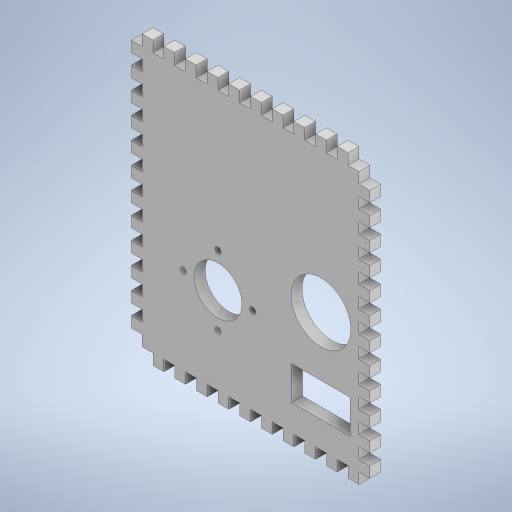
# Autodesk Inventor part: topside
Saved by Autodesk Inventor 2024 (Build 280153000, 153)
## iProperties
Created: 2024-04-15
Part Number: topside
Material: Generic
Document SubType Name: Modeling
Designer: srika
Density: 1 g/cm^3
Appearance: Default
Author: srika
Autodesk Inventor part; units mm, degrees
ref_plane "YZ Plane" through (0, 0, 0) normal (1, 0, 0) x (0, 1, 0)
ref_plane "XZ Plane" through (0, 0, 0) normal (0, 1, 0) x (-1, 0, 0)
ref_plane "XY Plane" through (0, 0, 0) normal (0, 0, 1) x (1, 0, 0)
sketch "Sketch1" plane through (0, 0, 0) normal (0, 0, 1) x (1, 0, 0)
  line L0 (5, 5) -> (105, 5)
  line L1 (105, 45) -> (105, 125)
  line L2 (105, 125) -> (5, 125)
  line L3 (5, 85) -> (5, 5)
  line L4 (0, 0) -> (5, 0)
  line L5 (5, 0) -> (5, 5)
  line L6 (5, 5) -> (0, 5)
  line L7 (0, 5) -> (0, 0)
  line L8 (105, 125) -> (110, 125)
  line L9 (110, 125) -> (110, 130)
  line L10 (110, 130) -> (105, 130)
  line L11 (105, 130) -> (105, 125)
  circle A0 centre (40, 45) radius 11
  circle A1 centre (24, 45) radius 1.4
  circle A2 centre (56, 45) radius 1.4
  circle A3 centre (40, 61) radius 1.4
  circle A4 centre (40, 29) radius 1.4
  circle A5 centre (87.5, 60) radius 13.7926
  line L12 (7.75, 7) -> (72.25, 7)
  line L13 (72.25, 7) -> (72.25, 83)
  line L14 (72.25, 83) -> (7.75, 83)
  line L15 (7.75, 83) -> (7.75, 7)
  line L16 (7.75, 7) -> (72.25, 83) construction
  line L17 (72.25, 7) -> (7.75, 83) construction
  line L18 (74, 17.25) -> (101, 17.25)
  line L19 (101, 17.25) -> (101, 32.75)
  line L20 (101, 32.75) -> (74, 32.75)
  line L21 (74, 32.75) -> (74, 17.25)
  line L22 (74, 17.25) -> (101, 32.75) construction
  line L23 (101, 17.25) -> (74, 32.75) construction
  line L24 (5, 125) -> (5, 85)
  line L25 (105, 45) -> (105, 5)
  line L26 (5, 15) -> (0, 15)
  line L27 (0, 10) -> (5, 10)
  line L28 (0, 15) -> (0, 10)
  line L29 (5, 10) -> (5, 15)
  line L30 (5, 25) -> (0, 25)
  line L31 (0, 20) -> (5, 20)
  line L32 (0, 25) -> (0, 20)
  line L33 (5, 20) -> (5, 25)
  line L34 (5, 35) -> (0, 35)
  line L35 (0, 30) -> (5, 30)
  line L36 (0, 35) -> (0, 30)
  line L37 (5, 30) -> (5, 35)
  line L38 (5, 45) -> (0, 45)
  line L39 (0, 40) -> (5, 40)
  line L40 (0, 45) -> (0, 40)
  line L41 (5, 40) -> (5, 45)
  line L42 (5, 55) -> (0, 55)
  line L43 (0, 50) -> (5, 50)
  line L44 (0, 55) -> (0, 50)
  line L45 (5, 50) -> (5, 55)
  line L46 (5, 65) -> (0, 65)
  line L47 (0, 60) -> (5, 60)
  line L48 (0, 65) -> (0, 60)
  line L49 (5, 60) -> (5, 65)
  line L50 (5, 75) -> (0, 75)
  line L51 (0, 70) -> (5, 70)
  line L52 (0, 75) -> (0, 70)
  line L53 (5, 70) -> (5, 75)
  line L54 (5, 85) -> (0, 85)
  line L55 (0, 80) -> (5, 80)
  line L56 (0, 85) -> (0, 80)
  line L57 (5, 80) -> (5, 85)
  line L58 (5, 95) -> (0, 95)
  line L59 (0, 90) -> (5, 90)
  line L60 (0, 95) -> (0, 90)
  line L61 (5, 90) -> (5, 95)
  line L62 (5, 105) -> (0, 105)
  line L63 (0, 100) -> (5, 100)
  line L64 (0, 105) -> (0, 100)
  line L65 (5, 100) -> (5, 105)
  line L66 (5, 115) -> (0, 115)
  line L67 (0, 110) -> (5, 110)
  line L68 (0, 115) -> (0, 110)
  line L69 (5, 110) -> (5, 115)
  line L70 (5, 125) -> (0, 125)
  line L71 (0, 120) -> (5, 120)
  line L72 (0, 125) -> (0, 120)
  line L73 (5, 120) -> (5, 125)
  line L74 (10, 0) -> (15, 0)
  line L75 (15, 0) -> (15, 5)
  line L76 (15, 5) -> (10, 5)
  line L77 (10, 5) -> (10, 0)
  line L78 (20, 0) -> (25, 0)
  line L79 (25, 0) -> (25, 5)
  line L80 (25, 5) -> (20, 5)
  line L81 (20, 5) -> (20, 0)
  line L82 (30, 0) -> (35, 0)
  line L83 (35, 0) -> (35, 5)
  line L84 (35, 5) -> (30, 5)
  line L85 (30, 5) -> (30, 0)
  line L86 (40, 0) -> (45, 0)
  line L87 (45, 0) -> (45, 5)
  line L88 (45, 5) -> (40, 5)
  line L89 (40, 5) -> (40, 0)
  line L90 (50, 0) -> (55, 0)
  line L91 (55, 0) -> (55, 5)
  line L92 (55, 5) -> (50, 5)
  line L93 (50, 5) -> (50, 0)
  line L94 (60, 0) -> (65, 0)
  line L95 (65, 0) -> (65, 5)
  line L96 (65, 5) -> (60, 5)
  line L97 (60, 5) -> (60, 0)
  line L98 (70, 0) -> (75, 0)
  line L99 (75, 0) -> (75, 5)
  line L100 (75, 5) -> (70, 5)
  line L101 (70, 5) -> (70, 0)
  line L102 (80, 0) -> (85, 0)
  line L103 (85, 0) -> (85, 5)
  line L104 (85, 5) -> (80, 5)
  line L105 (80, 5) -> (80, 0)
  line L106 (90, 0) -> (95, 0)
  line L107 (95, 0) -> (95, 5)
  line L108 (95, 5) -> (90, 5)
  line L109 (90, 5) -> (90, 0)
  line L110 (100, 0) -> (105, 0)
  line L111 (105, 0) -> (105, 5)
  line L112 (105, 5) -> (100, 5)
  line L113 (100, 5) -> (100, 0)
  line L114 (105, 120) -> (105, 115)
  line L115 (110, 120) -> (105, 120)
  line L116 (110, 115) -> (110, 120)
  line L117 (105, 115) -> (110, 115)
  line L118 (105, 110) -> (105, 105)
  line L119 (110, 110) -> (105, 110)
  line L120 (110, 105) -> (110, 110)
  line L121 (105, 105) -> (110, 105)
  line L122 (105, 100) -> (105, 95)
  line L123 (110, 100) -> (105, 100)
  line L124 (110, 95) -> (110, 100)
  line L125 (105, 95) -> (110, 95)
  line L126 (105, 90) -> (105, 85)
  line L127 (110, 90) -> (105, 90)
  line L128 (110, 85) -> (110, 90)
  line L129 (105, 85) -> (110, 85)
  line L130 (105, 80) -> (105, 75)
  line L131 (110, 80) -> (105, 80)
  line L132 (110, 75) -> (110, 80)
  line L133 (105, 75) -> (110, 75)
  line L134 (105, 70) -> (105, 65)
  line L135 (110, 70) -> (105, 70)
  line L136 (110, 65) -> (110, 70)
  line L137 (105, 65) -> (110, 65)
  line L138 (105, 60) -> (105, 55)
  line L139 (110, 60) -> (105, 60)
  line L140 (110, 55) -> (110, 60)
  line L141 (105, 55) -> (110, 55)
  line L142 (105, 50) -> (105, 45)
  line L143 (110, 50) -> (105, 50)
  line L144 (110, 45) -> (110, 50)
  line L145 (105, 45) -> (110, 45)
  line L146 (105, 40) -> (105, 35)
  line L147 (110, 40) -> (105, 40)
  line L148 (110, 35) -> (110, 40)
  line L149 (105, 35) -> (110, 35)
  line L150 (105, 30) -> (105, 25)
  line L151 (110, 30) -> (105, 30)
  line L152 (110, 25) -> (110, 30)
  line L153 (105, 25) -> (110, 25)
  line L154 (105, 20) -> (105, 15)
  line L155 (110, 20) -> (105, 20)
  line L156 (110, 15) -> (110, 20)
  line L157 (105, 15) -> (110, 15)
  line L158 (105, 10) -> (105, 5)
  line L159 (110, 10) -> (105, 10)
  line L160 (110, 5) -> (110, 10)
  line L161 (105, 5) -> (110, 5)
  line L162 (95, 130) -> (95, 125)
  line L163 (100, 130) -> (95, 130)
  line L164 (100, 125) -> (100, 130)
  line L165 (95, 125) -> (100, 125)
  line L166 (85, 130) -> (85, 125)
  line L167 (90, 130) -> (85, 130)
  line L168 (90, 125) -> (90, 130)
  line L169 (85, 125) -> (90, 125)
  line L170 (75, 130) -> (75, 125)
  line L171 (80, 130) -> (75, 130)
  line L172 (80, 125) -> (80, 130)
  line L173 (75, 125) -> (80, 125)
  line L174 (65, 130) -> (65, 125)
  line L175 (70, 130) -> (65, 130)
  line L176 (70, 125) -> (70, 130)
  line L177 (65, 125) -> (70, 125)
  line L178 (55, 130) -> (55, 125)
  line L179 (60, 130) -> (55, 130)
  line L180 (60, 125) -> (60, 130)
  line L181 (55, 125) -> (60, 125)
  line L182 (45, 130) -> (45, 125)
  line L183 (50, 130) -> (45, 130)
  line L184 (50, 125) -> (50, 130)
  line L185 (45, 125) -> (50, 125)
  line L186 (35, 130) -> (35, 125)
  line L187 (40, 130) -> (35, 130)
  line L188 (40, 125) -> (40, 130)
  line L189 (35, 125) -> (40, 125)
  line L190 (25, 130) -> (25, 125)
  line L191 (30, 130) -> (25, 130)
  line L192 (30, 125) -> (30, 130)
  line L193 (25, 125) -> (30, 125)
  line L194 (15, 130) -> (15, 125)
  line L195 (20, 130) -> (15, 130)
  line L196 (20, 125) -> (20, 130)
  line L197 (15, 125) -> (20, 125)
  line L198 (5, 130) -> (5, 125)
  line L199 (10, 130) -> (5, 130)
  line L200 (10, 125) -> (10, 130)
  line L201 (5, 125) -> (10, 125)
  point P0 (87.5, 25)
  point P1 (7.75, 17)
  point P2 (7.75, 27)
  point P3 (7.75, 37)
  point P4 (7.75, 47)
  point P5 (7.75, 57)
  point P6 (7.75, 67)
  point P7 (7.75, 77)
  point P8 (7.75, 87)
  point P9 (7.75, 97)
  point P10 (7.75, 107)
  point P11 (7.75, 117)
  point P12 (7.75, 127)
  point P13 (105, 115)
  point P14 (105, 105)
  point P15 (105, 95)
  point P16 (105, 85)
  point P17 (105, 75)
  point P18 (105, 65)
  point P19 (105, 55)
  point P20 (105, 35)
  point P21 (105, 25)
  point P22 (105, 15)
  point P23 (95, 125)
  point P24 (85, 125)
  point P25 (75, 125)
  point P26 (65, 125)
  point P27 (55, 125)
  point P28 (45, 125)
  point P29 (35, 125)
  point P30 (25, 125)
  point P31 (15, 125)
  point P32 (5, 125)
  dimension "d0" = 100
  dimension "d1" = 80
  dimension "d16" = 5
  dimension "d17" = 5
  dimension "d32" = 22
  dimension "d33" = 2.8
  dimension "d34" = 2.8
  dimension "d35" = 2.8
  dimension "d36" = 2.8
  dimension "d39" = 10
  dimension "d46" = 10
  dimension "d53" = 10
  dimension "d60" = 10
  constraints: 400 end point, 90 horizontal alignment, 49 parallel, 40 collinear, 6 centre point, 5 vertical, 4 horizontal, 4 midpoint, 4 perpendicular, 222 other
  measures "d0" distance of L24.start L8.start
  measures "d1" distance of L1.end L1.start
  measures "d16" distance of L10.end L9.end
  measures "d17" distance of L9.end L8.end
  measures "d32" diameter of A0
  measures "d33" diameter of A1
  measures "d34" diameter of A2
  measures "d35" diameter of A3
  measures "d36" diameter of A4
  measures "d39" distance of L3.end L26.start
  measures "d46" distance of L3.end L75.end
  measures "d53" distance of L8.start L114.end
  measures "d60" distance of L10.end L162.start
extrude "Extrusion1" add sketch "Sketch1" along normal blind 5 contours L3 L24 L2 L1 L25 L0 | L0 L75 L74 L77 | L27 L28 L26 L3 | L0 L79 L78 L81 | L31 L32 L30 L3 | L0 L83 L82 L85 | L35 L36 L34 L3 | L0 L87 L86 L89 | L39 L40 L38 L3 | L0 L91 L90 L93 | L43 L44 L42 L3 | L0 L95 L94 L97 | L47 L48 L46 L3 | L0 L99 L98 L101 | L51 L52 L50 L3 | L0 L103 L102 L105 | L55 L56 L54 L3 | L0 L107 L106 L109 | L59 L60 L58 L24 | L0 L111 L110 L113 | L63 L64 L62 L24 | L25 L159 L160 L161 | L67 L68 L66 L24 | L25 L155 L156 L157 | L71 L72 L70 L24 | L25 L151 L152 L153 | L198 L199 L200 L2 | L25 L147 L148 L149 | L194 L195 L196 L2 | L1 L143 L144 L145 | L190 L191 L192 L2 | L1 L139 L140 L141 | L186 L187 L188 L2 | L1 L135 L136 L137 | L182 L183 L184 L2 | L1 L131 L132 L133 | L178 L179 L180 L2 | L1 L127 L128 L129 | L174 L175 L176 L2 | L1 L123 L124 L125 | L170 L171 L172 L2 | L1 L119 L120 L121 | L166 L167 L168 L2 | L1 L115 L116 L117 | L162 L163 L164 L2 | L15 L14 L13 L12
body "Solid1"
